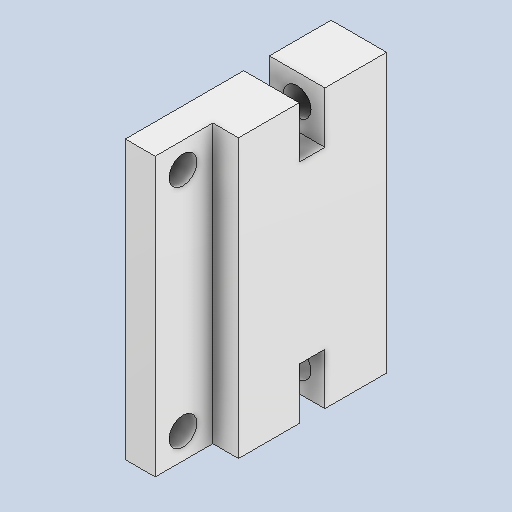
# Autodesk Inventor part: Vertical_Connector
Saved by Autodesk Inventor 2024.3 (Build 283343000, 343)
## iProperties
Created: 2024-09-06
Part Number: Vertical_Connector
Material: LCP 플라스틱
Document SubType Name: Modeling
Designer: 구지현
Density: 1.626 g/cm^3
Appearance: 매끄러움 - 흰색
Author: 구지현
Autodesk Inventor part; units mm, degrees
ref_plane "YZ Plane" through (0, 0, 0) normal (1, 0, 0) x (0, 1, 0)
ref_plane "XZ Plane" through (0, 0, 0) normal (0, 1, 0) x (-1, 0, 0)
ref_plane "작업 평면1" through (-17.0116, -44.6019, 14.5) normal (0, 0, -1) x (0, 1, 0)
sketch "스케치4" plane through (0, 0, 0) normal (0, 0, 1) x (1, 0, 0)
  arc A0 (-34.0751, 6.2636) -> (-34.5943, 4.5766) centre (-31.5943, 4.5766) ccw projected
  line L0 (-34.5943, -39.6766) -> (-34.5943, 4.5766) projected
  arc A1 (-34.5943, -39.6766) -> (-34.0751, -41.3636) centre (-31.5943, -39.6766) ccw projected
  line L1 (-30.3872, -46.7869) -> (-34.0751, -41.3636) projected
  arc A2 (-30.3872, -46.7869) -> (-27.9064, -48.1) centre (-27.9064, -45.1) ccw projected
  line L2 (-1.0822, -48.1) -> (-27.9064, -48.1) projected
  arc A3 (-1.0822, -48.1) -> (1.3986, -46.7869) centre (-1.0822, -45.1) ccw projected
  line L3 (5.0865, -41.3636) -> (1.3986, -46.7869) projected
  arc A4 (5.0865, -41.3636) -> (5.6057, -39.6766) centre (2.6057, -39.6766) ccw projected
  line L4 (5.6057, 4.5766) -> (5.6057, -39.6766) projected
  arc A5 (5.6057, 4.5766) -> (5.0865, 6.2636) centre (2.6057, 4.5766) ccw projected
  line L5 (1.1009, 12.1246) -> (5.0865, 6.2636) projected
  arc A6 (1.1009, 12.1246) -> (-0.5529, 13) centre (-0.5529, 11) ccw projected
  line L6 (-6.8443, 13) -> (-0.5529, 13) projected
  arc A7 (-5.3443, 11.5) -> (-6.8443, 13) centre (-6.8443, 11.5) ccw projected
  line L7 (-5.3443, 11.5) -> (-5.3443, 10) projected
  arc A8 (-5.3443, 10) -> (-2.9943, 7.65) centre (-2.9943, 10) ccw projected
  line L8 (-2.9943, 7.65) -> (-0.9943, 7.65) projected
  arc A9 (0.0057, 6.65) -> (-0.9943, 7.65) centre (-0.9943, 6.65) ccw projected
  line L9 (0.0057, 6.65) -> (0.0057, -36.15) projected
  arc A10 (-0.9943, -37.15) -> (0.0057, -36.15) centre (-0.9943, -36.15) ccw projected
  line L10 (-0.9943, -37.15) -> (-2.9943, -37.15) projected
  arc A11 (-2.9943, -37.15) -> (-5.3443, -39.5) centre (-2.9943, -39.5) ccw projected
  line L11 (-5.3443, -39.5) -> (-5.3443, -41.5) projected
  arc A12 (-6.3443, -42.5) -> (-5.3443, -41.5) centre (-6.3443, -41.5) ccw projected
  line L12 (-6.3443, -42.5) -> (-22.6443, -42.5) projected
  arc A13 (-23.6443, -41.5) -> (-22.6443, -42.5) centre (-22.6443, -41.5) ccw projected
  line L13 (-23.6443, -41.5) -> (-23.6443, -39.5) projected
  arc A14 (-23.6443, -39.5) -> (-25.9943, -37.15) centre (-25.9943, -39.5) ccw projected
  line L14 (-25.9943, -37.15) -> (-27.9943, -37.15) projected
  arc A15 (-28.9943, -36.15) -> (-27.9943, -37.15) centre (-27.9943, -36.15) ccw projected
  line L15 (-28.9943, -36.15) -> (-28.9943, 6.65) projected
  arc A16 (-27.9943, 7.65) -> (-28.9943, 6.65) centre (-27.9943, 6.65) ccw projected
  line L16 (-27.9943, 7.65) -> (-25.9943, 7.65) projected
  arc A17 (-25.9943, 7.65) -> (-23.6443, 10) centre (-25.9943, 10) ccw projected
  line L17 (-23.6443, 10) -> (-23.6443, 11.5) projected
  arc A18 (-22.1443, 13) -> (-23.6443, 11.5) centre (-22.1443, 11.5) ccw projected
  line L18 (-28.4357, 13) -> (-22.1443, 13) projected
  arc A19 (-28.4357, 13) -> (-30.0896, 12.1246) centre (-28.4357, 11) ccw projected
  line L19 (-34.0751, 6.2636) -> (-30.0896, 12.1246) projected
  circle A20 centre (2.8057, 4) radius 1.35 projected
  circle A21 centre (2.8057, -18) radius 1.35 projected
  circle A22 centre (-3.4943, -45.3) radius 1.35 projected
  circle A23 centre (-31.7943, 4) radius 1.35 projected
  circle A24 centre (-31.7943, -18) radius 1.35 projected
  circle A25 centre (-25.4943, -45.3) radius 1.35 projected
  circle A26 centre (2.8057, -40) radius 1.35 projected
  circle A27 centre (-31.7943, -40) radius 1.35 projected
  line L20 (-31.7943, -40) -> (-31.7943, -18)
  line L21 (-29.0943, -15.5) -> (-34.4943, -15.5)
  line L22 (-34.4943, -15.5) -> (-34.4943, -42.5)
  line L23 (-34.4943, -42.5) -> (-29.0943, -42.5)
  line L24 (-29.0943, -42.5) -> (-29.0943, -15.5)
  line L25 (-29.0943, -15.5) -> (-34.4943, -42.5) construction
  line L26 (-34.4943, -15.5) -> (-29.0943, -42.5) construction
  point P0 (0, 0)
  point P1 (-31.7943, -29)
  dimension "d10" = 5.4
  dimension "d11" = 27
  constraints: 14 end point, 3 midpoint, 2 parallel, 1 horizontal, 1 perpendicular, 1 vertical
  measures "d10" distance of L23.end L22.end
  measures "d11" distance of L22.end L21.end
extrude "돌출4" add sketch "스케치4" against normal blind 6 contours L22 L21 L24 L23 L1 A1 | A1 L1 L23 L22
sketch "스케치5" plane through (0, 0, 0) normal (0, 0, 1) x (1, 0, 0)
  line L0 (-34.4943, -15.5) -> (-34.4943, -42.5) projected
  line L1 (-34.4943, -42.5) -> (-29.0943, -42.5) projected
  line L2 (-29.0943, -42.5) -> (-29.0943, -15.5) projected
  line L3 (-29.0943, -15.5) -> (-34.4943, -15.5) projected
  circle A0 centre (-31.7943, -40) radius 1.35 projected
  circle A1 centre (-31.7943, -18) radius 1.35 projected
  point P0 (0, 0)
extrude "돌출5" add sketch "스케치5" along normal blind 14.4 contours L3 L2 L1 L0 | A0 | A1
sketch "스케치6" plane through (-34.4943, -42.5, -6) normal (-1, 0, 0) x (0, 0, 1)
  line L0 (25.6, 57) -> (29.1, 57) projected
  line L1 (25.6, 57) -> (20.5, 51) projected
  line L2 (20.5, 51) -> (20.5, -2.1) projected
  line L3 (20.5, -2.1) -> (25.6, -8.1) projected
  line L4 (25.6, -8.1) -> (55.6, -8.1) projected
  line L5 (55.6, -8.1) -> (60.7, -2.1) projected
  line L6 (60.7, -2.1) -> (60.7, 51) projected
  line L7 (60.7, 51) -> (55.6, 57) projected
  line L8 (52.1, 57) -> (55.6, 57) projected
  arc A0 (55.1, 54) -> (52.1, 57) centre (52.1, 54) ccw projected
  line L9 (55.1, 0.5) -> (55.1, 54) projected
  arc A1 (52.1, -2.5) -> (55.1, 0.5) centre (52.1, 0.5) ccw projected
  line L10 (29.1, -2.5) -> (52.1, -2.5) projected
  arc A2 (26.1, 0.5) -> (29.1, -2.5) centre (29.1, 0.5) ccw projected
  line L11 (26.1, 54) -> (26.1, 0.5) projected
  arc A3 (29.1, 57) -> (26.1, 54) centre (29.1, 54) ccw projected
  circle A4 centre (57.9, 46.5) radius 1.35 projected
  circle A5 centre (57.9, 24.5) radius 1.35 projected
  circle A6 centre (57.9, 2.5) radius 1.35 projected
  circle A7 centre (51.6, -5.3) radius 1.35 projected
  circle A8 centre (23.3, 46.5) radius 1.35 projected
  circle A9 centre (23.3, 24.5) radius 1.35 projected
  circle A10 centre (23.3, 2.5) radius 1.35 projected
  circle A11 centre (29.6, -5.3) radius 1.35 projected
  line L12 (20.4, 27) -> (0, 27) projected
  line L13 (0, 0) -> (0, 27) projected
  line L14 (0, 0) -> (20.4, 0) projected
  line L15 (20.4, 27) -> (20.4, 0) projected
  line L16 (20.4, 0) -> (20.4, 27)
  line L17 (20.4, 27) -> (26, 27)
  line L18 (26, 27) -> (26, 0)
  line L19 (26, 0) -> (20.4, 0)
  point P0 (6, 42.5)
  dimension "d16" = 5.6
  constraints: 8 end point, 3 parallel, 1 perpendicular
  measures "d16" distance of L12.start L17.end
extrude "돌출6" add sketch "스케치6" against normal blind 2.9 contours L17 L18 L19 L2 | L2 L19 L15 L17
sketch "스케치7" plane through (-34.4943, -42.5, -6) normal (-1, 0, 0) x (0, 0, 1)
  line L0 (0, 1.15) -> (0, 3.85) projected
  line L1 (6, 3.85) -> (6, 1.15) projected
  line L2 (0, 23.15) -> (0, 25.85) projected
  line L3 (0, 23.15) -> (0, 25.85) projected
  line L4 (6, 2.5) -> (0, 2.5)
  line L5 (0, 2.5) -> (0, 24.5)
  line L6 (0, 24.5) -> (6, 24.5)
  line L7 (6, 24.5) -> (6, 2.5)
  line L8 (6, 2.5) -> (6, 24.5)
  line L9 (6, 24.5) -> (7.25, 24.5)
  line L10 (7.25, 24.5) -> (7.25, 2.5)
  line L11 (7.25, 2.5) -> (6, 2.5)
  line L12 (8.5, 5) -> (6, 5)
  line L13 (6, 5) -> (6, 0)
  line L14 (6, 0) -> (8.5, 0)
  line L15 (8.5, 0) -> (8.5, 5)
  line L16 (8.5, 5) -> (6, 0) construction
  line L17 (6, 5) -> (8.5, 0) construction
  line L18 (8.5, 22) -> (6, 22)
  line L19 (6, 22) -> (6, 27)
  line L20 (6, 27) -> (8.5, 27)
  line L21 (8.5, 27) -> (8.5, 22)
  line L22 (8.5, 22) -> (6, 27) construction
  line L23 (6, 22) -> (8.5, 27) construction
  point P0 (6, 42.5)
  point P1 (6, 5)
  point P2 (6, 1.15)
  dimension "d19" = 1.25
  dimension "d20" = 2.5
  dimension "d21" = 5
  dimension "d22" = 2.5
  dimension "d23" = 5
  constraints: 40 end point, 8 parallel, 6 midpoint, 5 perpendicular, 3 horizontal
  measures "d19" distance of L6.end L9.end
  measures "d20" distance of L14.end L13.end
  measures "d21" distance of L13.end L12.end
  measures "d22" distance of L19.end L20.end
  measures "d23" distance of L18.end L19.end
extrude "돌출7" cut sketch "스케치7" against normal through all contours L11 L10 L12 L15 L14 L13 L1 | L1 L7 L12 L10 L11 | L9 L10 L18 L7 | L19 L20 L21 L18 L10 L9
move faces "이동1" translate (0, 0, 6) faces at (-29.5959, -25.5425, -6) (-32.6943, -37.5, 1.6667) (-32.6943, -20.5, 0.8333) (-30.8943, -17.1667, 2.5) (-29.5443, -18, 0) (-30.4487, -18.1086, -4) (-30.8943, -15.5, -2) (-30.8943, -39.1667, 2.5) (-29.5443, -40, 0) (-30.4487, -40.1086, -4) (-32.6943, -42.5, -4)
